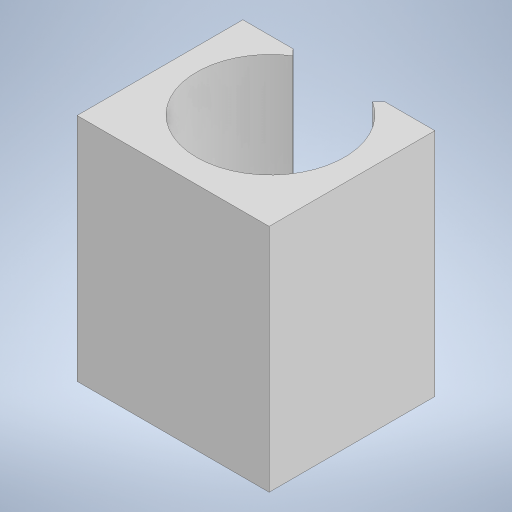
# Autodesk Inventor part: SBR20_BearingBlock
Saved by Autodesk Inventor 2024 (Build 280153000, 153)
## iProperties
Created: 2023-11-20
Part Number: SBR20_BearingBlock
Material: Generic
Document SubType Name: Modeling
Designer: KirikDK
Density: 1 g/cm^3
Appearance: Default
Author: KirikDK
Autodesk Inventor part; units mm, degrees
ref_plane "YZ Plane" through (0, 0, 0) normal (1, 0, 0) x (0, 1, 0)
ref_plane "XZ Plane" through (0, 0, 0) normal (0, 1, 0) x (-1, 0, 0)
ref_plane "XY Plane" through (0, 0, 0) normal (0, 0, 1) x (1, 0, 0)
sketch "Sketch1" plane through (0, 0, 0) normal (0, 1, 0) x (-1, 0, 0)
  line L0 (-23.54, 18.8125) -> (-23.54, -4.7733)
  line L1 (-23.54, 18.8125) -> (-23.54, 29.166)
  line L2 (-23.54, 29.166) -> (22.1671, 29.166)
  line L3 (22.1671, 29.166) -> (22.1671, -6.834)
  line L4 (18.6136, -6.834) -> (20.1065, -6.834)
  line L5 (22.1671, -4.7733) -> (22.1671, 18.8125)
  line L6 (-22.4793, 29.166) -> (21.1065, 29.166)
  line L7 (-23.54, 18.8125) -> (-23.54, -6.834)
  line L8 (-23.54, -6.834) -> (22.1671, -6.834)
  circle A0 centre (-0.6864, 8.0196) radius 16.05
  line L9 (-23.54, 29.166) -> (22.1671, 29.166)
  line L10 (22.1671, 29.166) -> (22.1671, 20.7196)
  line L11 (22.1671, 20.7196) -> (-23.54, 20.7196)
  line L12 (-23.54, 20.7196) -> (-23.54, 29.166)
  circle A1 centre (-0.6864, -15) radius 12.8668
  point P0 (0, 0)
  point P1 (7.98, -5.4895)
  point P2 (9.257, -6.834)
  point P3 (22.1671, 20.7196)
  point P4 (-23.54, 20.7196)
  point P5 (-23.54, -4.7733)
  point P6 (-10.6298, -6.834)
  point P7 (-9.3528, -5.4895)
  dimension "d0" = 0
  dimension "d1" = 32.1
  dimension "d2" = 0
  dimension "d3" = 0
  constraints: 26 end point, 2 centre point, 2 parallel, 2 perpendicular, 2 point on line, 2 vertical, 1 coincident, 1 horizontal
  measures "d0" distance between parallel lines of L6 L2
  measures "d1" diameter of A0
  measures "d2" distance between parallel lines of L3 L10
  measures "d3" distance between parallel lines of L7 L12
extrude "Extrusion1" add sketch "Sketch1" along normal blind 50 contours L1 L11 A0 A1 L8 L7 L0 | L1 L2 L3 L11 A0 | L11 L3 L8 L4 A1 A0
sketch "Sketch5" plane through (0, 50, 0) normal (0, 1, 0) x (1, 0, 0)
  line L0 (23.54, -29.166) -> (23.54, 6.834) projected
  line L1 (23.54, 6.834) -> (21.54, 6.834)
  line L2 (21.54, 6.834) -> (21.54, -29.166)
  line L3 (21.54, -29.166) -> (23.54, -29.166)
  line L4 (23.54, -29.166) -> (23.54, 6.834)
  line L5 (-22.1671, 6.834) -> (-22.1671, -29.166) projected
  line L6 (-22.1671, 6.834) -> (-20.1671, 6.834)
  line L7 (-20.1671, 6.834) -> (-20.1671, -29.166)
  line L8 (-20.1671, -29.166) -> (-22.1671, -29.166)
  line L9 (-22.1671, -29.166) -> (-22.1671, 6.834)
  point P0 (0, 0)
  dimension "d16" = 2
  dimension "d17" = 2
  constraints: 16 end point, 4 parallel, 2 horizontal, 2 perpendicular, 1 point on line
  measures "d16" distance of L5.start L6.end
  measures "d17" distance of L0.end L1.end
extrude "Extrusion3" cut sketch "Sketch5" against normal blind 100
body "Solid1"
